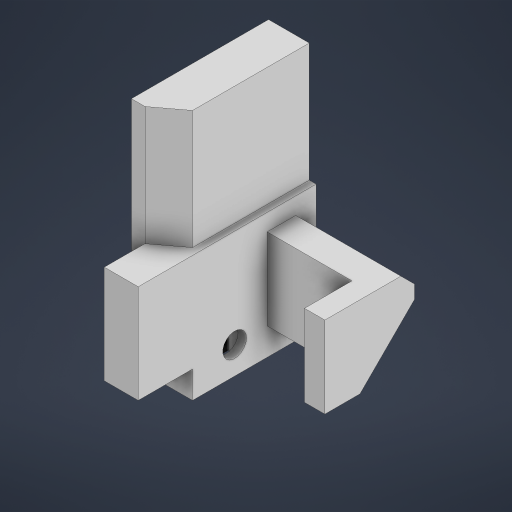
# Autodesk Inventor part: motor halterrung
Saved by Autodesk Inventor 2024.2 (Build 282272000, 272)
## iProperties
Created: 2024-02-26
Part Number: motor halterrung
Material: Generisch
Document SubType Name: Modeling
Designer: jacob
Density: 1 g/cm^3
Appearance: Vorgabe
Author: jacob
Autodesk Inventor part; units mm, degrees
ref_plane "YZ Plane" through (0, 0, 0) normal (1, 0, 0) x (0, 1, 0)
ref_plane "XZ Plane" through (0, 0, 0) normal (0, 1, 0) x (-1, 0, 0)
ref_plane "XY Plane" through (0, 0, 0) normal (0, 0, 1) x (1, 0, 0)
sketch "Skizze1" plane through (0, 0, 0) normal (0, 1, 0) x (-1, 0, 0)
  line L0 (0, 0) -> (-3, 0)
  line L1 (-3, 0) -> (-3, -10)
  line L2 (-3, -10) -> (19.5, -10)
  line L3 (12.5, -7) -> (0, -7)
  line L4 (0, -7) -> (0, 0)
  line L5 (12.5, -7) -> (12.5, 4)
  line L6 (12.5, 4) -> (19.5, 4)
  line L7 (19.5, 4) -> (19.5, -10)
  dimension "d0" = 12.5
  dimension "d1" = 3
  dimension "d2" = 3
  dimension "d3" = 7
  dimension "d4" = 11
  dimension "d5" = 7
  constraints: 16 end point, 5 perpendicular, 1 horizontal, 1 vertical
  measures "d0" distance of L3.start L3.end
  measures "d1" distance of L0.start L0.end
  measures "d2" distance between parallel lines of L2 L3
  measures "d3" distance between parallel lines of L7 L5
  measures "d4" distance of L3.start L5.end
  measures "d5" distance of L3.end L0.start
extrude "Extrusion1" add sketch "Skizze1" along normal blind 8
sketch "Skizze2" plane through (0, 0, 0) normal (0, -1, 0) x (1, 0, 0)
  line L0 (-12.5, 4) -> (-17.5, 4)
  line L1 (-17.5, 4) -> (-17.5, -8)
  line L2 (-17.5, -8) -> (-12.5, -8)
  line L3 (-12.5, -8) -> (-12.5, 4)
  point P0 (0, 0)
  point P1 (-19.5, -8)
  dimension "d14" = 5
  constraints: 8 end point, 2 parallel, 1 horizontal, 1 perpendicular, 1 point on line
  measures "d14" distance of L2.end L1.end
extrude "Extrusion2" add sketch "Skizze2" along normal blind 8
sketch "Skizze3" plane through (-17.5, 0, -8) normal (-1, 0, 0) x (0, 0, 1)
  line L0 (-2, 0) -> (12, 0) projected
  line L1 (12, 0) -> (12, -8) projected
  point P0 (8, 0)
  point P1 (5.793, -4)
  point P2 (0, 0)
  dimension "d17" = 4
  dimension "d18" = 6.207
  measures "d17" distance from line of L0 point (5.793, -4)
  measures "d18" distance from line of L1 point (5.793, -4)
hole "Bohrung1" at (-17.5, -4, -2.207) direction (1, 0, 0) diameter 3.5 end through all
sketch "Skizze4" plane through (0, -8, 0) normal (0, -1, 0) x (1, 0, 0)
  line L0 (-16.25, 0.593) -> (-13.75, 0.593)
  line L1 (-13.75, 0.593) -> (-13.75, -5.007)
  line L2 (-13.75, -5.007) -> (-16.25, -5.007)
  line L3 (-16.25, -5.007) -> (-16.25, 0.593)
  line L4 (-12.5, 4) -> (-17.5, 4) projected
  point P0 (0, 0)
  point P1 (-15, 0.593)
  point P2 (-15, 4)
  point P3 (-16.25, -2.207)
  dimension "d26" = 5.6
  dimension "d27" = 2.5
  dimension "d28" = 6.207
  constraints: 8 end point, 3 midpoint, 2 parallel, 1 horizontal, 1 perpendicular, 1 vertical alignment
  measures "d26" distance of L0.end L1.end
  measures "d27" distance of L1.end L2.end
  measures "d28" distance from line of L4 point (-16.25, -2.207)
extrude "Extrusion3" cut sketch "Skizze4" against normal blind 7
sketch "Skizze5" plane through (-19.5, 8, 4) normal (0, 0, 1) x (1, 0, 0)
  line L0 (7, -16) -> (7, 0) projected
  line L1 (2, -8) -> (2, -16) projected
  line L2 (7, 0) -> (2, 0)
  line L3 (2, 0) -> (2, -12)
  line L4 (2, -12) -> (7, -12)
  line L5 (7, -12) -> (7, 0)
  point P0 (19.5, -8)
  dimension "d31" = 12
  constraints: 8 end point, 2 parallel, 1 horizontal, 1 midpoint, 1 perpendicular
  measures "d31" distance between parallel lines of L2 L4
extrude "Extrusion4" add sketch "Skizze5" along normal blind 8
sketch "Skizze6" plane through (0, 8, 0) normal (0, 1, 0) x (1, 0, 0)
  line L0 (-12.5, 7) -> (-12.5, -12) projected
  line L1 (-12.5, 7) -> (-12.5, 8)
  line L2 (-19.5, 8) -> (1, 8) projected
  line L3 (-19.5, 10) -> (-19.5, -4) projected
  line L4 (-19.5, -4) -> (-17.5, -4) projected
  line L5 (-17.5, -4) -> (-17.5, -12) projected
  line L6 (-12.5, -12) -> (-17.5, -12) projected
  line L7 (-12.5, 7) -> (-12.5, -12) projected
  line L8 (-12.5, 7) -> (0, 7) projected
  line L9 (0, 7) -> (0, 0) projected
  line L10 (0, 0) -> (3, 0) projected
  line L11 (-12.5, 8) -> (-19.5, 8)
  line L12 (-19.5, 8) -> (-19.5, -4)
  line L13 (-17.5, -4) -> (-19.5, -4)
  line L14 (-17.5, -4) -> (-17.5, -12)
  line L15 (-12.5, -12) -> (-17.5, -12)
  line L16 (-17.5, -6) -> (-12.5, -6)
  line L17 (3, 0) -> (3, 10) projected
  line L18 (3, 10) -> (-19.5, 10) projected
  line L19 (-13.5, -6) -> (-13.5, 8)
  line L20 (-13.5, -6) -> (-13.5, -12)
  point P0 (-19.5, 8)
  point P1 (-13.5, 8)
  dimension "d39" = 14
  dimension "d70" = 1
  constraints: 18 end point, 6 point on line, 5 perpendicular, 2 collinear, 1 vertical
  measures "d39" distance between parallel lines of L11 L16
  measures "d70" distance between parallel lines of L19 L0
extrude "Extrusion6" add sketch "Skizze6" along normal blind 2.5 contours L20 L6 L5 L16
extrude "Extrusion7" add sketch "Skizze6" along normal blind 20 contours L16 L5 L4 L3 L2 L19
sketch "Skizze9" plane through (0, 28, 0) normal (0, 1, 0) x (1, 0, 0)
  line L0 (-17.5, -6) -> (-13.5, -6) projected
  line L1 (-17.5, -6) -> (-19.5, -6)
  line L2 (-19.5, -4) -> (-17.5, -4) projected
  line L3 (-19.5, -6) -> (-19.5, -4)
  line L4 (-17.5, -4) -> (-17.5, -6) projected
  line L5 (-17.5, -4) -> (-17.5, -6)
  line L6 (-19.5, 8) -> (-19.5, -4) projected
  line L7 (-17.5, -4) -> (-19.5, -4)
  point P0 (0, 0)
  point P1 (-12.5, -7)
  constraints: 8 end point, 2 horizontal, 1 collinear, 1 perpendicular, 1 other
extrude "Extrusion8" add sketch "Skizze9" against normal up to surface (28 mm away)
chamfer "Fasen4" distance 4 distance2 3 1 edges at (-13.5, 19.25, 6) measured on face at (-14, 19.25, 6)
sketch "Skizze10" plane through (3, 0, -10) normal (0, 0, -1) x (-1, 0, 0)
  line L0 (15.5, 0) -> (20.5, 0) projected
  line L1 (15.5, 0) -> (15.5, -8) projected
  line L2 (20.5, -8) -> (15.5, -8) projected
  line L3 (20.5, 0) -> (20.5, -8) projected
  line L4 (15.5, 0) -> (20.5, 0) projected
  line L5 (15.5, 0) -> (15.5, 8)
  line L6 (22.5, 8) -> (15.5, 8)
  line L7 (22.5, 0) -> (22.5, 8) projected
  line L8 (22.5, 8) -> (22.5, 0)
  line L9 (22.5, 0) -> (15.5, 0)
  line L10 (0, 0) -> (22.5, 0) projected
  line L11 (22.5, 0) -> (22.5, 8) projected
  line L12 (0, 8) -> (22.5, 8) projected
  line L13 (0, 0) -> (0, 8) projected
  line L14 (22.5, 8) -> (16.5, 8) projected
  line L15 (22.5, 8) -> (22.5, 28) projected
  line L16 (16.5, 28) -> (22.5, 28) projected
  line L17 (16.5, 8) -> (16.5, 28) projected
  point P0 (3, 0)
  constraints: 8 end point, 3 perpendicular, 1 collinear
extrude "Extrusion9" add sketch "Skizze10" along normal blind 4.2 contours L5 L6 L7 L9 L0
sketch "Skizze12" plane through (-12.5, 0, -8) normal (0, 0, -1) x (-1, 0, 0)
  line L0 (0, 0) -> (5, 0) projected
  line L1 (0, 0) -> (0, -8) projected
  line L2 (5, -8) -> (0, -8) projected
  line L3 (5, 0) -> (5, -8) projected
  point P0 (-12.5, 0)
extrude "Extrusion10" add sketch "Skizze12" along normal up to surface (6.2 mm away)
chamfer "Fasen8" distance 2 angle 45 1 edges at (-18.5, 0, -14.2)
chamfer "Fasen9" distance 4 angle 45 1 edges at (-18.5, 0, 6)
sketch "Skizze13" plane through (-13.5, 8, -8) normal (0, 0, -1) x (-1, 0, 0)
  line L0 (6, 0) -> (0, 0) projected
  line L1 (6, 0) -> (6, 20) projected
  line L2 (0, 20) -> (6, 20) projected
  line L3 (0, 0) -> (0, 20) projected
  point P0 (-13.5, -8)
extrude "Extrusion11" add sketch "Skizze13" along normal up to surface (6.2 mm away)
sketch "Skizze14" plane through (0, 8, 0) normal (0, 1, 0) x (1, 0, 0)
  line L0 (-13.5, 14.2) -> (-13.5, -12) projected
  line L1 (-12.5, -12) -> (-13.5, -12) projected
  line L2 (-12.5, 7) -> (-12.5, -12) projected
  line L3 (-12.5, 7) -> (0, 7) projected
  line L4 (0, 7) -> (0, 0) projected
  line L5 (0, 0) -> (3, 0) projected
  line L6 (3, 0) -> (3, 10) projected
  line L7 (-12.5, 10) -> (-12.5, 14.2) projected
  line L8 (-13.5, 14.2) -> (-12.5, 14.2) projected
  line L9 (-12.5, 7.5) -> (3, 7.5) projected
  line L10 (-12.5, 7.5) -> (-12.5, 7)
  line L11 (3, 10) -> (-12.5, 10) projected
  point P0 (3, 7.5)
  constraints: 2 end point, 1 perpendicular
extrude "Extrusion12" add sketch "Skizze14" along normal up to surface (2.5 mm away) contours L8 L7 L11 L6 L9 L10 L2 L1 L0
sketch "Skizze15" plane through (0, 0, 0) normal (0, -1, 0) x (1, 0, 0)
  line L0 (-12.5, -7) -> (-12.5, -10) projected
  line L1 (3, -10) -> (-12.5, -10) projected
  line L2 (3, 0) -> (3, -10) projected
  line L3 (0, 0) -> (3, 0) projected
  line L4 (0, -7) -> (0, 0) projected
  line L5 (-12.5, -7) -> (0, -7) projected
extrude "Extrusion13" add sketch "Skizze15" along normal blind 4
chamfer "Fasen10" distance 2 angle 45 1 edges at (-4.75, -4, -10)
sketch "Skizze17" plane through (3, 8, -7.5) normal (1, 0, 0) x (0, 0, -1)
  line L0 (2.5, -10) -> (2.5, 2.5) projected
  line L1 (2.5, 2.5) -> (0, 2.5) projected
  line L2 (0, 0) -> (0, 2.5) projected
  line L3 (-7.5, 0) -> (0, 0) projected
  line L4 (-7.5, -12) -> (-7.5, 0) projected
  line L5 (0.5, -12) -> (-7.5, -12) projected
  line L6 (2.5, -10) -> (0.5, -12) projected
  line L7 (0, 0) -> (2.5, 0)
  line L8 (2.5, -10) -> (2.5, 2.5) projected
  point P0 (-7.5, -8)
  point P1 (2.5, -2.5)
  constraints: 2 end point, 1 perpendicular, 1 point on line
extrude "Extrusion15" cut sketch "Skizze17" against normal up to surface (15.5 mm away) contours L7 L2 L1 L0
sketch "Skizze18" plane through (-12.5, -8, 4) normal (1, 0, 0) x (0, 0, -1)
  line L0 (14, 6) -> (14, 16) projected
  line L1 (14, 6) -> (17.2, 9.2)
  line L2 (17.2, 9.2) -> (17.2, 16)
  line L3 (17.2, 16) -> (14, 16)
  line L4 (12, 4) -> (14, 6) projected
  line L5 (18.2, 0) -> (18.2, 18.5) projected
  point P0 (4, 8)
  dimension "d87" = 1
  constraints: 6 end point, 1 collinear, 1 perpendicular, 1 vertical
  measures "d87" distance between parallel lines of L5 L2
extrude "Extrusion16" add sketch "Skizze18" along normal up to surface (15.5 mm away)
chamfer "Fasen12" distance 2 angle 45 1 edges at (-4.75, 8, -13.2)
chamfer "Fasen13" distance 2 angle 45 1 edges at (3, -1.4, -10.6)
